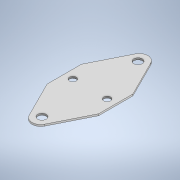
# Autodesk Inventor part: Platte2
Saved by Autodesk Inventor 2022 (Build 260153000, 153)
## iProperties
Created: 2022-04-02
Part Number: Platte2
Material: Generic
Document SubType Name: Modeling
Designer: benni
Density: 1 g/cm^3
Appearance: Default
Author: benni
Autodesk Inventor part; units mm, degrees
ref_plane "YZ Plane" through (0, 0, 0) normal (1, 0, 0) x (0, 1, 0)
ref_plane "XZ Plane" through (0, 0, 0) normal (0, 1, 0) x (-1, 0, 0)
ref_plane "XY Plane" through (0, 0, 0) normal (0, 0, 1) x (1, 0, 0)
sketch "Sketch1" plane through (0, 0, 0) normal (0, 1, 0) x (-1, 0, 0)
  line L0 (0, 0) -> (30, 0)
  line L1 (30, 0) -> (30, -20)
  line L2 (30, -20) -> (0, -20)
  line L3 (0, -20) -> (0, 0)
  line L4 (30, -10) -> (0, -10)
  line L5 (15, 0) -> (15, -20)
  circle A0 centre (25, -10) radius 2
  circle A1 centre (15, -38) radius 2.5
  line L6 (30, -20) -> (19.5, -41)
  circle A2 centre (5, -10) radius 2
  line L7 (0, -20) -> (10.5, -41)
  arc A3 (10.5, -41) -> (19.5, -41) centre (15, -38.75) ccw
  line L8 (30, 0) -> (0, 0)
  circle A4 centre (15, 18) radius 2.5
  line L9 (30, 0) -> (19.5, 21)
  line L10 (0, 0) -> (10.5, 21)
  arc A5 (19.5, 21) -> (10.5, 21) centre (15, 18.75) ccw
  dimension "d0" = 20
  dimension "d1" = 30
  dimension "d2" = 5
  dimension "d3" = 4
  dimension "d5" = 18
  dimension "d6" = 5
  dimension "d7" = 21
  dimension "d8" = 10.5
  constraints: 22 end point, 8 symmetric about line, 6 centre point, 4 midpoint, 4 point on circle, 3 coincident, 2 parallel, 1 horizontal, 1 perpendicular, 1 point on line, 1 tangent, 3 other
  measures "d0" distance of L0.end L1.end
  measures "d1" distance of L1.end L2.end
  measures "d2" distance from line of L1 point (25, -10)
  measures "d3" diameter of A0
  measures "d5" distance from line of L2 point (15, -38)
  measures "d6" diameter of A1
  measures "d7" distance from line of L2 L6.end
  measures "d8" distance from line of L1 L6.end
extrude "Extrusion1" add sketch "Sketch1" along normal blind 1 contours L10 A5 L9 L0 | L0 L5 L4 A2 L3 | L0 L1 L4 A0 L5 | L4 A2 L5 L2 L3 | L4 A0 L1 L2 L5 | L2 L6 A3 L7
body "Solid1"
